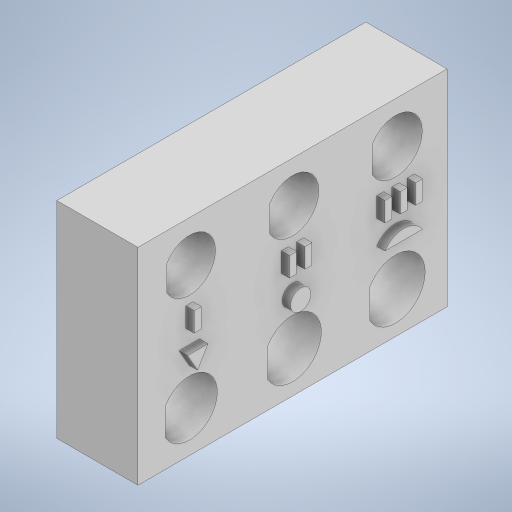
# Autodesk Inventor part: shaft hole tester
Saved by Autodesk Inventor 2023 (Build 270158000, 158)
## iProperties
Created: 2023-02-01
Part Number: shaft hole tester
Material: Generic
Document SubType Name: Modeling
Designer: Steven
Density: 1 g/cm^3
Appearance: Default
Author: Steven
Autodesk Inventor part; units mm, degrees
ref_plane "YZ Plane" through (0, 0, 0) normal (1, 0, 0) x (0, 1, 0)
ref_plane "XZ Plane" through (0, 0, 0) normal (0, 1, 0) x (-1, 0, 0)
ref_plane "XY Plane" through (0, 0, 0) normal (0, 0, 1) x (1, 0, 0)
sketch "Sketch1" plane through (0, 0, 0) normal (1, 0, 0) x (0, 1, 0)
  line L0 (12.7, 19.05) -> (-12.7, 19.05)
  line L1 (-12.7, 19.05) -> (-12.7, -19.05)
  line L2 (-12.7, -19.05) -> (12.7, -19.05)
  line L3 (12.7, -19.05) -> (12.7, 19.05)
  line L4 (12.7, 19.05) -> (-12.7, -19.05) construction
  line L5 (-12.7, 19.05) -> (12.7, -19.05) construction
  arc A0 (6.0166, 15.4771) -> (9.2234, 15.4771) centre (7.62, 12.7) ccw
  line L6 (6.0166, 15.4771) -> (9.2234, 15.4771)
  arc A1 (6.0008, 2.8046) -> (9.2393, 2.8046) centre (7.62, 0) ccw
  line L7 (6.0008, 2.8046) -> (9.2393, 2.8046)
  arc A2 (5.969, -9.8404) -> (9.271, -9.8404) centre (7.62, -12.7) ccw
  line L8 (5.969, -9.8404) -> (9.271, -9.8404)
  arc A3 (-9.3345, 15.6696) -> (-5.9055, 15.6696) centre (-7.62, 12.7) ccw
  line L9 (-9.3345, 15.6696) -> (-5.9055, 15.6696)
  arc A4 (-9.398, 3.0796) -> (-5.842, 3.0796) centre (-7.62, 0) ccw
  line L10 (-9.398, 3.0796) -> (-5.842, 3.0796)
  arc A5 (-9.4456, -9.5379) -> (-5.7944, -9.5379) centre (-7.62, -12.7) ccw
  line L11 (-9.4456, -9.5379) -> (-5.7944, -9.5379)
  line L12 (3.4886, 13.1373) -> (1.0834, 13.1373)
  line L13 (1.0834, 13.1373) -> (1.0834, 12.2627)
  line L14 (1.0834, 12.2627) -> (3.4886, 12.2627)
  line L15 (3.4886, 12.2627) -> (3.4886, 13.1373)
  line L16 (3.4886, 13.1373) -> (1.0834, 12.2627) construction
  line L17 (1.0834, 13.1373) -> (3.4886, 12.2627) construction
  line L18 (12.7, 0) -> (-12.7, 0) construction
  line L19 (3.4886, 1.3826) -> (1.0834, 1.3826)
  line L20 (1.0834, 1.3826) -> (1.0834, 0.508)
  line L21 (1.0834, 0.508) -> (3.4886, 0.508)
  line L22 (3.4886, 0.508) -> (3.4886, 1.3826)
  line L23 (3.4886, 1.3826) -> (1.0834, 0.508) construction
  line L24 (1.0834, 1.3826) -> (3.4886, 0.508) construction
  line L25 (3.4886, -0.508) -> (1.0834, -0.508)
  line L26 (1.0834, -0.508) -> (1.0834, -1.3826)
  line L27 (1.0834, -1.3826) -> (3.4886, -1.3826)
  line L28 (3.4886, -1.3826) -> (3.4886, -0.508)
  line L29 (3.4886, -0.508) -> (1.0834, -1.3826) construction
  line L30 (1.0834, -0.508) -> (3.4886, -1.3826) construction
  line L31 (1.0834, -13.1373) -> (3.4886, -13.1373)
  line L32 (3.4886, -12.2627) -> (1.0834, -12.2627)
  line L33 (1.0834, -12.2627) -> (1.0834, -13.1373)
  line L34 (3.4886, -13.1373) -> (3.4886, -12.2627)
  line L35 (3.4886, -12.2627) -> (1.0834, -13.1373) construction
  line L36 (1.0834, -12.2627) -> (3.4886, -13.1373) construction
  line L37 (1.0834, -15.0279) -> (3.4886, -15.0279)
  line L38 (3.4886, -14.1533) -> (1.0834, -14.1533)
  line L39 (1.0834, -14.1533) -> (1.0834, -15.0279)
  line L40 (3.4886, -15.0279) -> (3.4886, -14.1533)
  line L41 (3.4886, -14.1533) -> (1.0834, -15.0279) construction
  line L42 (1.0834, -14.1533) -> (3.4886, -15.0279) construction
  line L43 (3.4886, -10.3721) -> (1.0834, -10.3721)
  line L44 (1.0834, -10.3721) -> (1.0834, -11.2467)
  line L45 (1.0834, -11.2467) -> (3.4886, -11.2467)
  line L46 (3.4886, -11.2467) -> (3.4886, -10.3721)
  line L47 (3.4886, -10.3721) -> (1.0834, -11.2467) construction
  line L48 (1.0834, -10.3721) -> (3.4886, -11.2467) construction
  line L49 (-0.889, 13.97) -> (-0.889, 11.43)
  line L50 (-0.889, 11.43) -> (-3.0887, 12.7)
  line L51 (-3.0887, 12.7) -> (-0.889, 13.97)
  circle A6 centre (-1.905, 0) radius 1.27
  arc A7 (-1.905, -15.0279) -> (-1.905, -10.3721) centre (-3.4035, -12.7) ccw
  line L52 (-1.905, -10.3721) -> (-1.905, -15.0279)
  point P0 (0, 0)
  point P1 (2.286, 12.7)
  point P2 (0, 19.05)
  point P3 (2.286, 0.9453)
  point P4 (2.286, -0.9453)
  point P5 (2.286, -12.7)
  point P6 (2.286, -14.5906)
  point P7 (2.286, -10.8094)
  point P8 (2.286, -12.2627)
  point P9 (2.286, -11.2467)
  point P10 (-0.889, 12.7)
  point P11 (0, 0)
  dimension "d0" = 6.4135
  dimension "d1" = 3.2067
  dimension "d2" = 6.477
  dimension "d3" = 3.2385
  dimension "d4" = 6.604
  dimension "d5" = 3.302
  dimension "d6" = 6.858
  dimension "d7" = 3.429
  dimension "d8" = 7.112
  dimension "d9" = 3.556
  dimension "d10" = 7.3025
  dimension "d11" = 3.6513
  dimension "d12" = 38.1
  dimension "d13" = 6.35
  dimension "d14" = 6.35
  dimension "d15" = 5.08
  dimension "d16" = 25.4
  dimension "d17" = 5.08
  dimension "d18" = 0.8746
  dimension "d19" = 2.4052
  dimension "d20" = 2.286
  dimension "d21" = 0.8746
  dimension "d22" = 2.4052
  dimension "d23" = 0.8746
  dimension "d24" = 2.4052
  dimension "d25" = 0.508
  dimension "d26" = 0.508
  dimension "d27" = 0.8746
  dimension "d28" = 2.4052
  dimension "d29" = 0.8746
  dimension "d30" = 2.4052
  dimension "d31" = 0.8746
  dimension "d32" = 2.4052
  dimension "d33" = 1.016
  dimension "d35" = 1.016
  dimension "d36" = 2.54
  dimension "d38" = 2.54
  dimension "d39" = 2.54
  dimension "d40" = 0.889
  dimension "d41" = 2.54
  dimension "d42" = 1.905
  dimension "d43" = 4.6558
  dimension "d44" = 2.7685
  dimension "d45" = 5.6895
  dimension "d46" = 6.35
  constraints: 106 end point, 21 midpoint, 14 parallel, 14 point on circle, 13 horizontal, 9 vertical alignment, 8 centre point, 7 perpendicular, 6 horizontal alignment, 3 point on line, 2 vertical
  measures "d0" diameter of A0
  measures "d1" distance of L6.start L6.end
  measures "d2" diameter of A1
  measures "d3" distance of L7.start L7.end
  measures "d4" diameter of A2
  measures "d5" distance of L8.start L8.end
  measures "d6" diameter of A3
  measures "d7" distance of L9.start L9.end
  measures "d8" diameter of A4
  measures "d9" distance of L10.start L10.end
  measures "d10" diameter of A5
  measures "d11" distance of L11.start L11.end
  measures "d12" distance between parallel lines of L2 L0
  measures "d13" distance from line of L0 A0.centre
  measures "d14" distance from line of L2 A2.centre
  measures "d15" distance from line of L3 A2.centre
  measures "d16" distance of L0.start L0.end
  measures "d17" distance from line of L1 A5.centre
  measures "d18" distance of L12.end L13.end
  measures "d19" distance of L13.end L14.end
  measures "d20" horizontal distance of point (0, 19.05) point (2.286, 12.7)
  measures "d21" distance of L19.end L21.start
  measures "d22" distance of L21.start L21.end
  measures "d23" distance of L25.end L27.start
  measures "d24" distance of L27.start L27.end
  measures "d25" distance between parallel lines of L18 L25
  measures "d26" distance between parallel lines of L18 L21
  measures "d27" distance of L33.start L33.end
  measures "d28" distance of L33.end L36.end
  measures "d29" distance of L38.end L39.end
  measures "d30" distance of L39.end L42.end
  measures "d31" distance of L43.end L45.start
  measures "d32" distance of L45.start L45.end
  measures "d33" distance of point (2.286, -12.263) point (2.286, -11.247)
  measures "d35" distance between parallel lines of L31 L38
  measures "d36" distance of L49.start L49.end
  measures "d38" distance of L50.end L49.start
  measures "d39" distance of L49.end L50.end
  measures "d40" horizontal distance of point (0, 19.05) point (-0.889, 12.7)
  measures "d41" diameter of A6
  measures "d42" distance of point (0, 0) A6.centre
  measures "d43" distance of L52.end L52.start
  measures "d44" radius of A7
  measures "d45" distance of point (2.286, -12.7) A7.centre
  measures "d46" distance from line of L2 A7.centre
extrude "Extrusion1" add sketch "Sketch1" along normal blind 10
extrude "Extrusion2" add sketch "Sketch1" along normal blind 11 contours L15 L14 L13 L12 | L22 L21 L20 L19 | L28 L27 L26 L25 | L33 L32 L34 L31 | L39 L38 L40 L37 | L46 L45 L44 L43 | L49 L50 L51 | A6 | L52 A7
equation "\"d38\" = d36"
equation "\"d39\" = d36"
body "Solid1"
